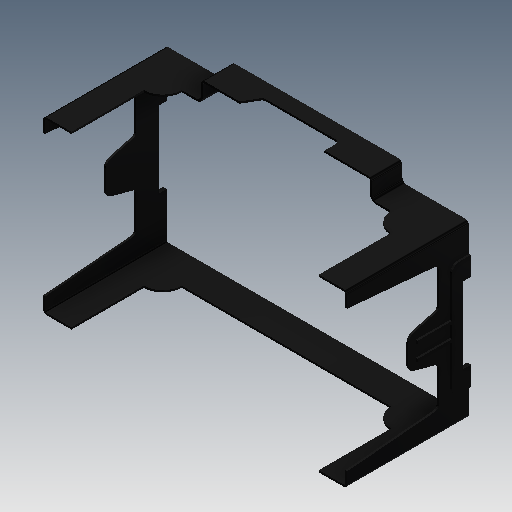
# Autodesk Inventor part: config - processor casing
Saved by Autodesk Inventor 2019.1 (Build 231200000, 200)
## iProperties
Company: Autodesk Asia Pte. Ltd.
Created: 2005-11-27
Part Number: config - processor casing
Document SubType Name: Modeling
Designer: Simon.Ng@autodesk.com
Stock Number: config - processor casing
Density: 1 g/cm^3
Material: Generic
Mass: 1.74352 g
Surface Area: 69.5144 cm^2
Volume: 1.74352 cm^3
Appearance: Glossy - Black
Title: PC Demo
Author: Simon.Ng@autodesk.com
Autodesk Inventor part; units mm, degrees
ref_plane "YZ Plane" through (0, 0, 0) normal (1, 0, 0) x (0, 1, 0)
ref_plane "XZ Plane" through (0, 0, 0) normal (0, 1, 0) x (-1, 0, 0)
ref_plane "XY Plane" through (0, 0, 0) normal (0, 0, 1) x (1, 0, 0)
sketch "Sketch1" plane through (0, 0, 0) normal (0, 0, 1) x (1, 0, 0)
  line L0 (0, 42.5) -> (0, -27.5) projected
  line L1 (-48, 0) -> (64, 0) projected
  line L2 (-40, 22.5) -> (40, 22.5)
  line L3 (40, 22.5) -> (40, -22.5)
  line L4 (40, -22.5) -> (-40, -22.5)
  line L5 (-40, -22.5) -> (-40, 22.5)
  line L6 (-22.5, 22.5) -> (22.5, 22.5)
  line L7 (22.5, 22.5) -> (22.5, 27.5)
  line L8 (22.5, 27.5) -> (-22.5, 27.5)
  line L9 (-22.5, 27.5) -> (-22.5, 22.5)
  dimension "d0" = 80
  dimension "d1" = 45
  dimension "d2" = 45
  dimension "d3" = 5
  constraints: 16 end point, 4 parallel, 2 horizontal, 2 perpendicular, 1 point on line, 3 other
  measures "d0" distance of L2.start L2.end
  measures "d1" distance of L4.end L2.start
  measures "d2" distance of L7.end L8.end
  measures "d3" distance of L8.end L6.start
extrude "Extrusion1" add sketch "Sketch1" along normal blind 32
fillet "Fillet2" radius 1 8 edges at (40, 22.5, 16) (40, -22.5, 16) (22.5, 22.5, 16) (22.5, 27.5, 16) (-22.5, 27.5, 16) (-22.5, 22.5, 16) (-40, 22.5, 16) (-40, -22.5, 16)
shell "Shell1" thickness 0.5 removed faces 2 at (7.6255, -7.4273, 32) at (7.6255, -7.4273, 0)
sketch "Sketch2" plane through (-40, -22.5, 0) normal (0, -1, 0) x (1, 0, 0)
  line L0 (80, 32) -> (0, 32) projected
  line L1 (0, 0) -> (80, 0) projected
  line L2 (80, 0) -> (80, 32) projected
  line L3 (7.5, 32) -> (7.5, 13)
  arc A0 (12.5, 8) -> (7.5, 13) centre (7.5, 8) ccw
  line L4 (12.5, 8) -> (67.5, 8)
  arc A1 (72.5, 13) -> (67.5, 8) centre (72.5, 8) ccw
  line L5 (72.5, 13) -> (72.5, 32)
  line L6 (7.5, 13) -> (24.0062, 13) construction
  line L7 (12.5, 8) -> (12.5, 12.4576) construction
  line L8 (72.5, 13) -> (51.974, 13) construction
  line L9 (67.5, 8) -> (67.5, 19.4272) construction
  line L10 (40, 41.6) -> (40, -3.2) construction
  dimension "d7" = 8
  dimension "d8" = 65
  dimension "d9" = 5
  constraints: 14 end point, 6 perpendicular, 4 point on circle, 4 tangent, 3 point on line, 2 centre point, 2 parallel, 1 symmetric about line, 2 other
  measures "d7" distance between parallel lines of L1 L4
  measures "d8" distance between parallel lines of L5 L3
  measures "d9" radius of A0
extrude "Extrusion2" cut sketch "Sketch2" against normal through all
sketch "Sketch3" plane through (40, -22.5, 0) normal (1, 0, 0) x (0, 0, -1)
  line L0 (-32, 45) -> (-32, 0) projected
  line L1 (0, 0) -> (0, 45) projected
  line L2 (0, 45) -> (-32, 45) projected
  line L3 (-41.6, 22.5) -> (3.2, 22.5) projected
  line L4 (-32, 41) -> (-8, 38.9003)
  line L5 (-8, 38.9003) -> (-8, 28.6436)
  line L6 (-8, 28.6436) -> (-16, 26.5)
  line L7 (-16, 26.5) -> (-16, 18.5)
  line L8 (-16, 18.5) -> (-8, 16.3564)
  line L9 (-8, 16.3564) -> (-8, 6.0997)
  line L10 (-8, 6.0997) -> (-32, 4)
  dimension "d12" = 8
  dimension "d13" = 4
  dimension "d14" = 95
  dimension "d15" = 8
  dimension "d16" = 8
  dimension "d17" = 105
  constraints: 14 end point, 2 parallel, 2 point on line, 2 symmetric about line, 1 perpendicular, 2 other
  measures "d12" distance between parallel lines of L1 L5
  measures "d13" distance from line of L2 L4.start
  measures "d14" angle of L4 L0
  measures "d15" distance of L6.end L7.end
  measures "d16" distance between parallel lines of L5 L7
  measures "d17" angle of L6 L5
extrude "Extrusion3" cut sketch "Sketch3" against normal through all contours L4 L5 L6 L7 L3 L0 | L3 L7 L8 L9 L10 L0
fillet "Fillet1" radius 2 4 edges at (-39.75, -4, 16) (-39.75, 4, 16) (39.75, -4, 16) (39.75, 4, 16)
fillet "Fillet1" radius 1 8 edges at (39.75, -6.1436, 8) (39.75, 6.1436, 8) (39.75, 16.4003, 8) (39.75, -16.4003, 8) (-39.75, -6.1436, 8) (-39.75, -16.4003, 8) (-39.75, 16.4003, 8) (-39.75, 6.1436, 8)
sketch "Sketch4" plane through (-21.5, 27.5, 0) normal (0, 1, 0) x (1, 0, 0)
  line L0 (0, -8) -> (43, -8) projected
  line L1 (21.5, 3.2) -> (21.5, -41.6) projected
  line L2 (9.1906, -8) -> (11.2113, -4.5)
  line L3 (12.0774, -4) -> (30.5, -4)
  line L4 (31.5, -5) -> (31.5, -8)
  arc A0 (12.0774, -4) -> (11.2113, -4.5) centre (12.0774, -5) ccw
  arc A1 (31.5, -5) -> (30.5, -4) centre (30.5, -5) ccw
  point P0 (11.5, -4)
  point P1 (31.5, -4)
  dimension "d23" = 4
  dimension "d24" = 120
  dimension "d25" = 20
  dimension "d26" = 1
  constraints: 6 end point, 6 point on line, 4 point on circle, 4 tangent, 2 centre point, 2 perpendicular, 1 equal radius, 1 symmetric about line
  measures "d23" distance of point (31.5, -4) L4.end
  measures "d24" angle of L3 L2
  measures "d25" distance of point (11.5, -4) point (31.5, -4)
  measures "d26" radius of A0
extrude "Extrusion4" cut sketch "Sketch4" against normal up to next
sketch "Sketch6" plane through (40, -21.5, 0) normal (1, 0, 0) x (0, 0, -1)
  arc A0 (-14.5176, 25.8972) -> (-16, 23.9653) centre (-14, 23.9653) ccw projected
  arc A1 (-16, 19.0347) -> (-14.5176, 17.1028) centre (-14, 19.0347) ccw projected
  line L0 (0, 0) -> (0, 43) projected
  line L1 (0, 36.5) -> (-3, 36.5)
  line L2 (-5, 34.5) -> (-5, 8.5)
  line L3 (-3, 6.5) -> (0, 6.5)
  line L4 (0, 6.5) -> (0, 36.5)
  line L5 (-41.6, 21.5) -> (3.2, 21.5) projected
  line L6 (-14, 23.9653) -> (-5, 23.9653)
  line L7 (-5, 23.9653) -> (-5, 23.1653)
  line L8 (-5, 23.1653) -> (-14, 23.1653)
  line L9 (-14, 23.1653) -> (-14, 23.9653)
  line L10 (-14, 19.0347) -> (-5, 19.0347)
  line L11 (-5, 19.0347) -> (-5, 19.8347)
  line L12 (-5, 19.8347) -> (-14, 19.8347)
  line L13 (-14, 19.8347) -> (-14, 19.0347)
  arc A2 (-3, 36.5) -> (-5, 34.5) centre (-3, 34.5) ccw
  arc A3 (-5, 8.5) -> (-3, 6.5) centre (-3, 8.5) ccw
  point P0 (-5, 6.5)
  point P1 (-5, 36.5)
  dimension "d29" = 5
  dimension "d30" = 30
  dimension "d31" = 0.8
  dimension "d32" = 2
  constraints: 24 end point, 7 point on line, 6 parallel, 4 point on circle, 4 tangent, 3 horizontal, 3 perpendicular, 2 centre point, 1 collinear, 1 equal radius, 1 other
  measures "d29" distance of L1.start point (-5, 36.5)
  measures "d30" distance of point (-5, 36.5) point (-5, 6.5)
  measures "d31" distance of L8.end L6.start
  measures "d32" radius of A2
extrude "Extrusion5" add sketch "Sketch6" along normal blind 0.5
sketch "Sketch7" plane through (40.5, -21.5, 0) normal (1, 0, 0) x (0, 0, -1)
  line L0 (0, 36.5) -> (0, 6.5) projected
  line L1 (-41.6, 21.5) -> (3.2, 21.5) projected
  line L2 (0, 31.5) -> (-2, 31.5)
  line L3 (-2, 31.5) -> (-2, 11.5)
  line L4 (-2, 11.5) -> (0, 11.5)
  line L5 (0, 11.5) -> (0, 31.5)
  dimension "d35" = 2
  dimension "d36" = 20
  constraints: 8 end point, 2 parallel, 1 horizontal, 1 perpendicular, 1 point on line, 1 other
  measures "d35" distance of L2.start L2.end
  measures "d36" distance of L2.end L3.end
extrude "Extrusion6" cut sketch "Sketch7" against normal up to next
mirror "Mirror1" about plane through (0, 0, 0) normal (1, 0, 0) of "Extrusion5", "Extrusion6"
body "Solid1"
